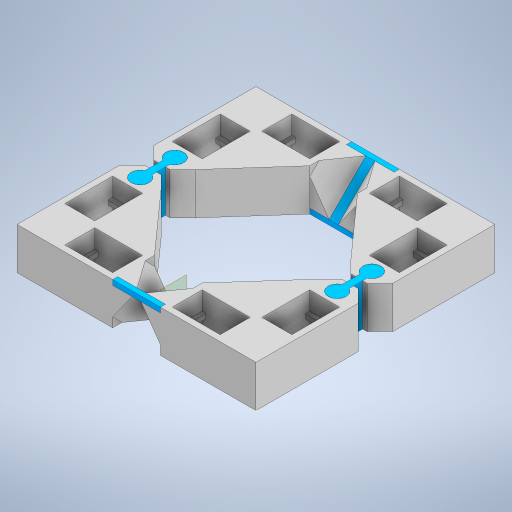
# Autodesk Inventor part: 6Bar_Bending_v2
Saved by Autodesk Inventor 2023 (Build 270158000, 158)
## iProperties
Created: 2022-07-18
Part Number: 6Bar_Bending_v2
Material: Generic
Document SubType Name: Modeling
Designer: hci-u
Density: 1 g/cm^3
Appearance: Default
Author: hci-u
Autodesk Inventor part; units mm, degrees
ref_plane "YZ Plane" through (0, 0, 0) normal (1, 0, 0) x (0, 1, 0)
ref_plane "XZ Plane" through (0, 0, 0) normal (0, 1, 0) x (-1, 0, 0)
sketch "Sketch1" plane through (0, 0, 0) normal (0, 1, 0) x (-1, 0, 0)
  line L0 (0, 0) -> (7, 0)
  line L1 (7, 0) -> (7, -7) construction
  line L2 (7, -7) -> (0, -7) construction
  line L3 (0, -7) -> (0, 0)
  line L4 (7, 0) -> (16, 0)
  line L5 (16, -7) -> (7, -7)
  line L6 (7, -7) -> (7, -17.1)
  line L7 (7, -17.1) -> (4.1, -20)
  line L8 (4.1, -20) -> (4.1, -17.1)
  line L9 (4.1, -17.1) -> (2.9, -17.1)
  line L10 (2.9, -17.1) -> (2.9, -20)
  line L11 (2.9, -20) -> (0, -17.1)
  line L12 (0, -17.1) -> (0, -7)
  line L13 (4.1, -20) -> (2.9, -20)
  line L14 (3.5, -17.1) -> (3.5, -20) construction
  line L15 (7, -17.1) -> (3.5, -17.1) construction
  line L16 (3.5, -17.1) -> (0, -17.1) construction
  line L17 (2.9, 0) -> (2.9, -20) construction
  line L18 (4.85, -19.25) -> (4.1, -19.25)
  line L19 (2.9, -19.25) -> (2.15, -19.25)
  line L20 (4.1, -20) -> (4.475, -19.25) construction
  line L21 (16, -7) -> (16, 0)
  line L22 (0, -3.5) -> (20, -3.5) construction
  line L23 (7, -17.1) -> (16, -7)
  circle A0 centre (3.5, -17.1) radius 1.5
  point P0 (2.9, -18.4748)
  point P1 (4.1, -18.4748)
  dimension "L_2" = 20
  dimension "wLink" = 7
  dimension "wFlex" = 1.2
  dimension "LenFlex" = 0.75
  dimension "LenDiagTPU" = 4
  dimension "d66" = 45
  dimension "d67" = 3
  constraints: 48 end point, 13 point on line, 7 equal length, 6 horizontal, 5 perpendicular, 4 midpoint, 2 coincident, 1 centre point, 1 collinear, 1 vertical, 6 other
  measures "L_2" distance between parallel lines of L0 L13
  measures "wLink" distance between parallel lines of L12 L6
  measures "wFlex" distance between parallel lines of L17 L8
  measures "LenFlex" distance from line of L7.end L18
  measures "LenDiagTPU" distance from line of L21 L22.end
  measures "d66" angle of L8 L7
  measures "d67" diameter of A0
extrude "Extrusion1" add sketch "Sketch1" along normal blind 7 contours L0 L4 L21 L5 L6 L7 L18 L8 A0 L10 L19 L11 L12 L3 | L23 L6 L5
ref_plane "Work Plane5" through (-20, 0, -7) normal (-1, 0, 0) x (0, 0, 1)
sketch "Sketch10" plane through (-16, 0, -7) normal (-1, 0, 0) x (0, 0, 1)
  line L0 (7, 7) -> (-10.1, 7) projected
  line L1 (7, 7) -> (6.1515, 7)
  line L2 (6.1515, 7) -> (0, 0.8485)
  line L3 (0, 0) -> (0.8485, 0)
  line L4 (7, 0) -> (-10.1, 0) projected
  line L5 (0.8485, 0) -> (7, 6.1515)
  line L6 (7, 0) -> (7, 7) projected
  line L7 (7, 7) -> (7, 6.1515)
  line L8 (0, 0) -> (0, 0.8485)
  line L9 (0, 0) -> (7, 7) construction
  line L10 (6.6551, 5.8065) -> (6.2308, 6.2308) construction
  line L11 (5.8065, 6.6551) -> (6.2308, 6.2308) construction
  dimension "d64" = 1.2
  constraints: 18 end point, 7 point on line, 4 parallel, 3 perpendicular, 1 collinear
  measures "d64" distance between parallel lines of L5 L2
extrude "Extrusion9" add sketch "Sketch10" along normal blind 4 contours L6 L5 L3 L8 L2 L0
chamfer "Chamfer1" distance 3.25 distance2 3.25 1 edges at (-16, 3.0757, -3.0757) measured on face at (-16, 2.0505, -2.0505)
chamfer "Chamfer2" distance 3.25 distance2 3.25 1 edges at (-16, 3.9243, -3.9243) measured on face at (-16, 4.9495, -4.9495)
sketch "Sketch11" plane through (-20, 0, -7) normal (-1, 0, 0) x (0, 0, 1)
  line L0 (7, 7) -> (-10.1, 7) projected
  line L1 (7, 0) -> (7, 7) projected
  line L2 (7, 7) -> (7, 6.1515)
  line L3 (0.8485, 0) -> (7, 6.1515) projected
  line L4 (7, 6.1515) -> (0.8485, 0)
  line L5 (-10.1, 0) -> (0, 0) projected
  line L6 (0.8485, 0) -> (0, 0)
  line L7 (0, 0.8485) -> (0, 0) projected
  line L8 (0, 0) -> (0, 0.8485)
  line L9 (6.1515, 7) -> (0, 0.8485) projected
  line L10 (0, 0.8485) -> (6.1515, 7)
  line L11 (6.1515, 7) -> (7, 7)
  constraints: 12 end point, 4 collinear, 1 parallel, 1 vertical
extrude "Extrusion10" cut sketch "Sketch11" against normal blind 4
mirror "Mirror1" about plane through (-20, 0, -7) normal (-1, 0, 0) of "Extrusion1", "Extrusion9", "Chamfer1", "Chamfer2", "Extrusion10"
sketch "Sketch15" plane through (0, 7, 0) normal (0, 1, 0) x (1, 0, 0)
  line L0 (0, 17.1) -> (-2.9, 20) construction
  line L1 (0, 17.1) -> (-2.15, 19.25) projected
  line L2 (-2.9, 19.25) -> (-2.9, 18.4748) construction
  line L3 (-2.9, 20) -> (-2.9, 17.1) construction
  constraints: 4 end point, 1 collinear, 1 vertical
ref_plane "Work Plane10" through (-16, 0, -20) normal (0, 0, 1) x (1, 0, 0)
mirror "Mirror2" about plane through (-16, 0, -20) normal (0, 0, 1) of "Extrusion1", "Mirror1", "Extrusion9", "Chamfer1", "Chamfer2", "Extrusion10"
sketch "Sketch6" plane through (0, 0, 0) normal (0, -1, 0) x (1, 0, 0)
  line L0 (-2.9, -20) -> (-4.1, -20)
  line L1 (-4.1, -20) -> (-4.1, -17.1)
  line L2 (-4.1, -17.1) -> (-2.9, -17.1)
  line L3 (-2.9, -17.1) -> (-2.9, -20)
  line L4 (-4.1, -18.4748) -> (-4.1, -19.25) projected
  line L5 (-4.1, -19.25) -> (-4.85, -19.25) projected
  line L6 (-2.9, -19.25) -> (-2.9, -18.4748) projected
  line L7 (-3.5, -22.9) -> (-3.5, -17.1) construction
  circle A0 centre (-3.5, -17.1) radius 1.5
  arc A1 (-4.1, -21.5252) -> (-2.9, -21.5252) centre (-3.5, -22.9) ccw projected
  arc A2 (-2.9, -18.4748) -> (-4.1, -18.4748) centre (-3.5, -17.1) ccw projected
  point P0 (0, 0)
  point P1 (-5, -1.8)
  point P2 (-5, -2.2)
  point P3 (-3.5, -20)
  point P4 (-2.9, -18.4748)
  point P5 (-4.1, -18.4748)
  constraints: 10 end point, 4 coincident, 3 midpoint, 2 collinear, 2 concentric, 2 parallel, 1 centre point, 1 horizontal, 1 perpendicular, 1 vertical
extrude "Extrusion5" add sketch "Sketch6" against normal up to surface (7 mm away) separate body
sketch "Sketch12" plane through (-16, 0, -7) normal (-1, 0, 0) x (0, 0, 1)
  line L0 (7, 7) -> (7, 6.1515) projected
  line L1 (7, 7) -> (7, 6.1515)
  line L2 (7, 6.1515) -> (0.8485, 0)
  line L3 (0, 0.8485) -> (6.1515, 7)
  line L4 (6.1515, 7) -> (7, 7)
  line L5 (0, 0) -> (0, 0.8485) projected
  line L6 (0.8485, 0) -> (0, 0)
  line L7 (0, 0) -> (0, 0.8485)
  line L8 (0, 0.8485) -> (6.1515, 7) projected
  line L9 (6.1515, 7) -> (7, 7) projected
  point P0 (7, 0)
  constraints: 12 end point, 2 collinear, 1 coincident, 1 horizontal, 1 perpendicular, 1 vertical
extrude "Extrusion11" add sketch "Sketch12" along normal blind 4 bodies 2
mirror "Mirror3" about plane through (-16, 0, -20) normal (0, 0, 1) of "Extrusion5", "Extrusion11" bodies 2
mirror "Mirror4" about plane through (-20, 0, -7) normal (-1, 0, 0) of "Extrusion5", "Mirror3", "Extrusion11" bodies 2
sketch "Sketch16" plane through (-16, 7, -40) normal (0, 1, 0) x (1, 0, 0)
  line L0 (10, -7) -> (15, -7)
  line L1 (15, -7) -> (15, -15)
  line L2 (15, -15) -> (10, -15)
  line L3 (10, -15) -> (10, -7)
  arc A0 (13.1, -18.4748) -> (11.9, -18.4748) centre (12.5, -17.1) ccw projected
  line L4 (12.5, -17.1) -> (12.5, -15) construction
  line L5 (16, 0) -> (0, 0) projected
  line L6 (9, -6) -> (1, -6)
  line L7 (1, -6) -> (1, -1)
  line L8 (1, -1) -> (9, -1)
  line L9 (9, -1) -> (9, -6)
  line L10 (16, 0) -> (16, -17.1) projected
  line L11 (12.5, -17.1) -> (16, -17.1) construction
  line L12 (1, -3.5) -> (9, -3.5) construction
  line L13 (5, -3.5) -> (5, 0) construction
  line L14 (12.5, -15) -> (12.5, 0) construction
  point P0 (16, -40)
  dimension "d68" = 5
  dimension "d70" = 8
  dimension "d75" = 7
  dimension "d85" = 5
  dimension "d86" = 8
  dimension "d87" = 7
  constraints: 26 end point, 5 perpendicular, 4 midpoint, 4 parallel, 2 horizontal, 2 point on line, 1 vertical
  measures "d68" distance between parallel lines of L1 L3
  measures "d70" distance between parallel lines of L2 L0
  measures "d75" distance between parallel lines of L5 L0
  measures "d85" distance between parallel lines of L8 L6
  measures "d86" distance between parallel lines of L9 L7
  measures "d87" distance between parallel lines of L10 L9
extrude "Extrusion14" cut sketch "Sketch16" against normal up to surface (7 mm away) bodies 1
sketch "Sketch17" plane through (0, 0, -22.9) normal (1, 0, 0) x (0, 0, -1)
  circle A0 centre (9.1, 3.5) radius 1
  line L0 (0, 0) -> (10.1, 0) projected
  line L1 (9.1, 0) -> (9.1, 3.5) construction
  line L2 (9.1, 3.5) -> (9.1, 7) construction
  line L3 (0, 7) -> (10.1, 7) projected
  line L4 (17.1, 0) -> (17.1, 7) projected
  point P0 (-22.9, 0)
  dimension "d73" = 2
  dimension "d74" = 8
  constraints: 4 end point, 3 point on line, 1 centre point, 1 collinear, 1 perpendicular
  measures "d73" diameter of A0
  measures "d74" distance from line of L4 L1.end
extrude "Extrusion15" [suppressed]
sketch "Sketch18" plane through (-6, 7, -25) normal (1, 0, 0) x (0, 0, -1)
  line L0 (0.7, -3.9) -> (0.7, -3.1)
  line L1 (0.7, -3.1) -> (0, -3.1)
  line L2 (8, -3.9) -> (7.3, -3.9)
  line L3 (7.3, -3.9) -> (7.3, -3.1)
  line L4 (7.3, -3.1) -> (8, -3.1)
  line L5 (8, -3.1) -> (8, -3.9)
  line L6 (0, 0) -> (8, 0) projected
  line L7 (4, 0) -> (4, -7) construction
  line L8 (0.7, -3.5) -> (4, -3.5) construction
  line L9 (7.3, -3.5) -> (4, -3.5) construction
  line L10 (8, 0) -> (8, -7) projected
  line L11 (0, -3.1) -> (0, -3.9)
  line L12 (0, 0) -> (0, -7) projected
  line L13 (0.7, -3.9) -> (0, -3.9)
  line L14 (8, -7) -> (0, -7) projected
  point P0 (-25, -7)
  dimension "d82" = 3.9
  dimension "d83" = 3.9
  dimension "d84" = 0.7
  constraints: 22 end point, 4 midpoint, 3 collinear, 3 equal length, 3 horizontal, 2 perpendicular, 2 point on line, 1 vertical
  measures "d82" distance between parallel lines of L14 L1
  measures "d83" distance between parallel lines of L6 L13
  measures "d84" distance between parallel lines of L12 L0
extrude "Extrusion16" add sketch "Sketch18" along normal up to surface (5 mm away) contours L13 L11 L1 L0 | L2 L3 L4 L5 bodies 1
sketch "Sketch20" plane through (-7, 7, -34) normal (0, 0, -1) x (-1, 0, 0)
  line L0 (0.6, -3.9) -> (0.6, -3.1)
  line L1 (0.6, -3.1) -> (0, -3.1)
  line L2 (8, -3.9) -> (7.4, -3.9)
  line L3 (7.4, -3.9) -> (7.4, -3.1)
  line L4 (7.4, -3.1) -> (8, -3.1)
  line L5 (8, -3.1) -> (8, -3.9)
  line L6 (0, 0) -> (8, 0) construction
  line L7 (4, 0) -> (4, -7.3559) construction
  line L8 (0.6, -3.5) -> (4, -3.5) construction
  line L9 (7.4, -3.5) -> (4, -3.5) construction
  line L10 (8, 0) -> (8, -7) construction
  line L11 (0, -3.1) -> (0, -3.9)
  line L12 (0, 0) -> (0, -7) construction
  line L13 (0.6, -3.9) -> (0, -3.9)
  line L14 (8, -7) -> (0, -7) construction
  line L15 (8, -7) -> (0, -7) projected
  line L16 (0, 0) -> (0, -7) projected
  line L17 (8, 0) -> (8, -7) projected
  point P0 (-7, -7)
  dimension "d88" = 3.9
  dimension "d89" = 3.9
  dimension "d90" = 0.6
  dimension "d91" = 0.8
  dimension "d92" = 3.5
  constraints: 28 end point, 5 collinear, 3 equal length, 3 horizontal, 3 midpoint, 3 point on line, 2 perpendicular, 1 vertical, 4 other
  measures "d89" distance between parallel lines of L6 L13
  measures "d90" distance between parallel lines of L12 L0
  measures "d91" distance of L0.start L0.end
  measures "d92" distance of the line from the sketch origin of L8
extrude "Extrusion17" add sketch "Sketch20" along normal up to surface (5 mm away) bodies 1
mirror "Mirror8" about plane through (-16, 0, -20) normal (0, 0, 1) of "Extrusion14", "Extrusion16", "Extrusion17" bodies 1
mirror "Mirror9" about plane through (-20, 0, -7) normal (-1, 0, 0) of "Extrusion14", "Mirror8", "Extrusion16", "Extrusion17" bodies 1
sketch "Sketch19" plane through (-16, 0, -40) normal (0, -1, 0) x (1, 0, 0)
  point P0 (16, 40)
sketch "Sketch7" plane through (0, 7, 0) normal (0, 1, 0) x (1, 0, 0)
  line L0 (0, 0) -> (-7, 0)
  line L1 (-7, 0) -> (-7, 40)
  line L2 (-7, 40) -> (0, 40)
  line L3 (0, 40) -> (0, 0)
  line L4 (-7, 17.1) -> (-7, 7) projected
  line L5 (0, 40) -> (-16, 40) projected
  point P0 (-40, 0)
  constraints: 8 end point, 2 collinear, 2 parallel, 1 horizontal, 1 perpendicular
sketch "Sketch8" plane through (0, 3.5, 0) normal (0, 1, 0) x (1, 0, 0)
  line L0 (-1.2, 5.2) -> (-2.8, 5.2)
  line L1 (-2.8, 5.2) -> (-2.8, 6.8)
  line L2 (-2.8, 6.8) -> (-1.2, 6.8)
  line L3 (-1.2, 6.8) -> (-1.2, 5.2)
  line L4 (-15, 0) -> (0, 0) projected
  line L5 (-2, 0) -> (-2, 5.2) construction
  line L6 (-1.2, 6) -> (0, 6) construction
  line L7 (0, 15) -> (0, 0) projected
  line L8 (-1.2, 33.421) -> (-2.8, 33.421)
  line L9 (-2.8, 33.421) -> (-2.8, 35.021)
  line L10 (-2.8, 35.021) -> (-1.2, 35.021)
  line L11 (-1.2, 35.021) -> (-1.2, 33.421)
  line L12 (-2, 35.021) -> (-3.5, 40) construction
  line L13 (-7, 40) -> (0, 40) projected
  line L14 (-21.2, 5.2) -> (-22.8, 5.2)
  line L15 (-22.8, 5.2) -> (-22.8, 6.8)
  line L16 (-22.8, 6.8) -> (-21.2, 6.8)
  line L17 (-21.2, 6.8) -> (-21.2, 5.2)
  line L18 (-21.2, 33.421) -> (-22.8, 33.421)
  line L19 (-22.8, 33.421) -> (-22.8, 35.021)
  line L20 (-22.8, 35.021) -> (-21.2, 35.021)
  line L21 (-21.2, 35.021) -> (-21.2, 33.421)
  line L22 (-20, 4) -> (-20, 0) projected
  line L23 (-21.8, 15) -> (-22.2, 15) projected
  line L24 (-22.8, 6) -> (-24, 6) construction
  line L25 (-24, 0) -> (-24, 9) projected
  dimension "d26" = 1.6
  dimension "d27" = 2
  dimension "d28" = 6
  dimension "d29" = 1.6
  constraints: 40 end point, 8 parallel, 7 equal length, 6 horizontal, 5 midpoint, 5 point on line, 4 perpendicular, 3 collinear, 1 vertical
  measures "d26" distance between parallel lines of L1 L3
  measures "d27" distance between parallel lines of L7 L5
  measures "d28" distance between parallel lines of L4 L6
  measures "d29" distance between parallel lines of L2 L0
sketch "Sketch9" plane through (0, 3.5, 0) normal (0, 1, 0) x (1, 0, 0)
  line L0 (-21, 5) -> (-23, 5)
  line L1 (-23, 5) -> (-23, 7)
  line L2 (-23, 7) -> (-21, 7)
  line L3 (-21, 7) -> (-21, 5)
  line L4 (-23, 35) -> (-21, 35)
  line L5 (-21, 33) -> (-23, 33)
  line L6 (-23, 33) -> (-23, 35)
  line L7 (-2.8, 33.2) -> (-1.2, 33.2) projected
  line L8 (-2.8, 5.2) -> (-2.8, 6.8) projected
  line L9 (-7, 15) -> (-7, 7) projected
  line L10 (-20, 9) -> (-20, 4) projected
  line L11 (-2.8, 5.2) -> (-1.2, 5.2) projected
  line L12 (-22, 5) -> (-22, 0) construction
  line L13 (-20, 0) -> (-24, 0) projected
  line L14 (-22.8, 6.8) -> (-21.2, 6.8) construction
  line L15 (-21.2, 6.8) -> (-21.2, 5.2) construction
  line L16 (-21.2, 5.2) -> (-22.8, 5.2) construction
  line L17 (-22.8, 5.2) -> (-22.8, 6.8) construction
  line L18 (-22, 5.2) -> (-22, 5) construction
  line L19 (-33, 33) -> (-25, 33) projected
  line L20 (-2.8, 33.2) -> (-2.8, 34.8) projected
  line L21 (-21, 35) -> (-21, 33)
  line L22 (-1.2, 6.8) -> (-1.2, 5.2) projected
  line L23 (-1.2, 6) -> (0, 6) construction
  line L24 (0, 0) -> (0, 15) projected
  line L25 (-1.2, 33.2) -> (-1.2, 34.8) projected
  line L26 (-1.2, 34) -> (0, 34) construction
  line L27 (0, 40) -> (0, 25) projected
  line L28 (-23, 34) -> (-24, 34) construction
  line L29 (-24, 15) -> (-24, 24) projected
  line L30 (-23, 6) -> (-24, 6) construction
  line L31 (-23, 6) -> (-22.8, 6) construction
  point P0 (-25, 33)
  dimension "d34" = 0.2
  constraints: 38 end point, 9 horizontal, 8 midpoint, 4 collinear, 4 equal length, 4 perpendicular, 4 point on line, 3 vertical, 2 parallel
  measures "d34" distance between parallel lines of L2 L14
sketch "Sketch13" plane through (0, 3.5, 0) normal (0, 1, 0) x (1, 0, 0)
  line L0 (-7, 40) -> (0, 33)
  line L1 (0, 40) -> (0, 25) projected
  line L2 (0, 33) -> (0, 40)
  line L3 (0, 40) -> (-7, 40)
  line L4 (-25, 40) -> (-40, 40) projected
  line L5 (-15, 0) -> (0, 0) projected
  line L6 (-40, 40) -> (0, 0) construction
  line L7 (-24, 0) -> (0, 40) construction
  point P0 (-15, 15)
  dimension "d58" = 45
  constraints: 10 end point, 3 point on line, 1 coincident, 1 vertical
  measures "d58" angle of L3 L0
ref_plane "Work Plane7" through (-1.8, 7, -20) normal (0, 0, -1) x (-1, 0, 0)
equation "\"d64\" = wFlex"
body "Solid1"
body "Solid2"
